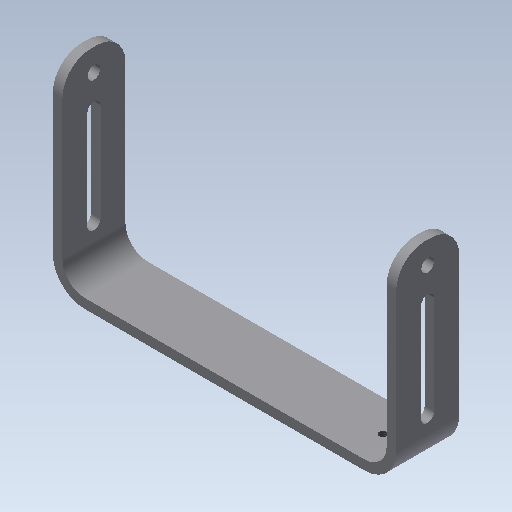
# Autodesk Inventor part: Haltegriff
Saved by Autodesk Inventor 2020.2 (Build 242310000, 310)
## iProperties
Created: 2014-03-25
Part Number: Haltegriff
Material: Generisch
Document SubType Name: Sheet Metal
Designer: schardt
Density: 1 g/cm^3
Flat Pattern Width: 1.98 cm
Flat Pattern Length: 22 cm
Flat Pattern Area: 43.56 cm^2
Sheet Metal Rule: Standard_mm
Sheet Metal Width: 19,800 mm
Sheet Metal Length: 220,000 mm
Sheet Metal Area: 4356,000 mm^2
Appearance: Vorgabe
Author: schardt
Autodesk Inventor part; units mm, degrees
ref_plane "YZ Plane" through (0, 0, 0) normal (1, 0, 0) x (0, 1, 0)
ref_plane "XZ Plane" through (0, 0, 0) normal (0, 1, 0) x (-1, 0, 0)
ref_plane "XY Plane" through (0, 0, 0) normal (0, 0, 1) x (1, 0, 0)
sketch "Skizze1" plane through (0, 0, 0) normal (0, 0, 1) x (1, 0, 0)
  line L0 (-110, -9.9) -> (110, -9.9)
  line L1 (110, -9.9) -> (110, 9.9)
  line L2 (110, 9.9) -> (-110, 9.9)
  line L3 (-110, 9.9) -> (-110, -9.9)
  line L4 (-110, -9.9) -> (110, 9.9) construction
  line L5 (110, -9.9) -> (-110, 9.9) construction
  point P0 (0, 0)
  dimension "d0" = 220
  dimension "d1" = 19.8
  measures "d0" distance of L2.end L1.end
  measures "d1" distance of L1.end L0.end
extrude "Grobblech1" add sketch "Skizze1" along normal blind 3
sketch "Skizze3" plane through (0, 0, 3) normal (0, 0, 1) x (1, 0, 0)
  line L0 (110, -9.9) -> (-110, -9.9) projected
  line L1 (-110, 9.9) -> (110, 9.9) projected
  line L2 (-44, -9.9) -> (-44, 9.9)
  line L3 (44, -9.9) -> (44, 9.9)
  point P0 (0, 0)
  dimension "d17" = 44
  dimension "d18" = 44
  constraints: 4 end point, 4 point on line, 2 perpendicular
  measures "d17" distance from line of point (0, 0) L2
  measures "d18" distance from line of point (0, 0) L3
fold "Falten3" angle 90 bend radius 7 thickness 3 k factor 0.44 line from (44, -9.9, 3) to (44, 9.9, 3) line at bend start moving side (1, 0, 0) folds toward (0, 0, 1)
fold "Falten4" angle 90 bend radius 7 thickness 3 k factor 0.44 line from (-44, -9.9, 3) to (-44, 9.9, 3) line at bend start moving side (-1, 0, 0) folds toward (0, 0, 1)
fillet "Eckenrundung1" radius 9 4 edges at (52.5, -9.9, 62.931) (52.5, 9.9, 62.931) (-52.5, 9.9, 62.931) (-52.5, -9.9, 62.931)
sketch "Skizze4" plane through (54, -9.9, 10) normal (1, 0, 0) x (0, 0, -1)
  line L0 (-52.931, 9) -> (-52.931, 10.8) projected
  line L1 (0, 0) -> (-43.931, 0) projected
  point P0 (10, 9.9)
  point P1 (-45.931, 9.9)
  dimension "d32" = 9.9
  dimension "d33" = 7
  measures "d32" distance from line of L1 point (-45.931, 9.9)
  measures "d33" distance from line of point (-45.931, 9.9) L0
hole "Bohrung1" at (54, 0, 55.931) direction (-1, 0, 0) diameter 4 end through all
sketch "Skizze5" plane through (54, -9.9, 10) normal (1, 0, 0) x (0, 0, -1)
  line L0 (0, 0) -> (-43.931, 0) projected
  line L1 (-3, 9.9) -> (-38, 9.9) construction
  line L2 (-5.1, 7.8) -> (-35.9, 7.8)
  line L3 (-35.9, 12) -> (-5.1, 12)
  arc A0 (-5.1, 7.8) -> (-5.1, 12) centre (-5.1, 9.9) ccw
  arc A1 (-35.9, 12) -> (-35.9, 7.8) centre (-35.9, 9.9) ccw
  point P0 (10, 9.9)
  point P1 (-20.5, 9.9)
  dimension "d41" = 9.9
  dimension "d42" = 13
  dimension "d43" = 4.2
  dimension "d44" = 35
  constraints: 8 end point, 6 point on circle, 4 tangent, 2 centre point, 2 parallel, 2 point on line, 1 midpoint
  measures "d41" distance between parallel lines of L0 L1
  measures "d42" distance of L1.start point (10, 9.9)
  measures "d43" distance between parallel lines of L2 L3
  measures "d44" distance of L1.end L1.start
extrude "Ausklinkung1" cut sketch "Skizze5" against normal through all
sketch "Skizze6" plane through (0, 0, 0) normal (0, 0, -1) x (-1, 0, 0)
  point P0 (0, 0)
  point P1 (-40, 0)
  dimension "d47" = 40
  constraints: 1 horizontal alignment
  measures "d47" distance of point (-40, 0) point (0, 0)
hole "Bohrung2" at (40, 0, 0) direction (0, 0, 1) diameter 2.459 end through all thread size "M3x0.5" class "6H" standard "ISO Metric profile"
equation "\"d19\" = BreiteBiegungsfreistellung"
equation "\"d20\" = TiefeBiegungsfreistellung"
equation "\"d21\" = MinimalRest"
equation "\"d22\" = Biegeradius"
equation "\"d55\" = Stärke"
equation "\"d25\" = BreiteBiegungsfreistellung"
equation "\"d26\" = TiefeBiegungsfreistellung"
equation "\"d27\" = MinimalRest"
equation "\"d28\" = Biegeradius"
equation "\"d39\" = Stärke"
equation "\"d45\" = Stärke"
equation "\"d53\" = Stärke"
equation "\"Biegeradius\" = Stärke"
equation "\"BreiteBiegungsfreistellung\" = Stärke"
equation "\"TiefeBiegungsfreistellung\" = 0.5 * Stärke"
equation "\"GrößeEckenfreistellung\" = 4 * Stärke"
equation "\"MinimalRest\" = 2 * Stärke"
equation "\"Übergangsradius\" = Biegeradius"
equation "\"JacobiRadiusGröße\" = Biegeradius"
equation "\"Abstandsgröße\" = Stärke"
equation "\"d2\" = Biegeradius"
equation "\"Stärke\" = 3"
